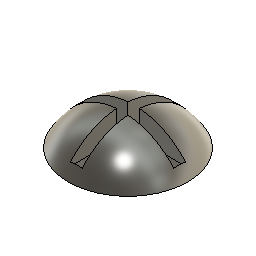
Screwhead (Autodesk Fusion 360 design; units mm, degrees)
Autodesk Fusion 360 part; units mm, degrees
sphere "SpherePrimitive1" add diameter 60 placed x (1, 0, 0) y (0, 1, 0) z (0, 0, 1) at (0, 0, 0)
sketch "Sketch2" plane through (0, 0, 0) normal (0, 0, 1) x (1, 0, 0)
  line L0 (22.5, 2.5) -> (22.5, -2.5)
  line L1 (2.5, 22.5) -> (-2.5, 22.5)
  line L2 (-22.5, 2.5) -> (-22.5, -2.5)
  line L3 (2.5, -22.5) -> (-2.5, -22.5)
  line L4 (-2.5, 22.5) -> (-2.5, 2.5)
  line L5 (-2.5, -2.5) -> (-2.5, -22.5)
  line L6 (-22.5, 2.5) -> (-2.5, 2.5)
  line L7 (2.5, 2.5) -> (22.5, 2.5)
  line L8 (2.5, 22.5) -> (2.5, 2.5)
  line L9 (2.5, -2.5) -> (2.5, -22.5)
  line L10 (-22.5, -2.5) -> (-2.5, -2.5)
  line L11 (2.5, -2.5) -> (22.5, -2.5)
  constraint collinear L4 L5
  constraint collinear L6 L7
  constraint coincident L9.start L10
  constraint collinear L8 L9
  constraint collinear L10 L11
extrude "Extrude1" cut sketch "Sketch2" along normal blind 45
sketch "Sketch3" plane through (0, -2.5, 0) normal (0, 1, 0) x (-1, 0, 0)
  arc A0 (-2.5, 29.7909) -> (-22.5, 19.685) centre (0, 0) ccw
  line L0 (-22.5, 19.685) -> (-22.5, 0)
  line L1 (-22.5, 0) -> (-2.5, 0)
  line L2 (-2.5, 0) -> (-2.5, 29.7909)
  line L3 (35, 15, -75) -> (-53.3891, 15, -75)
  line L4 (-53.3891, 15, -75) -> (-53.3891, -53.8167, -75)
  line L5 (-53.3891, -53.8167, -75) -> (35, -53.8167, -75)
  line L6 (35, -53.8167, -75) -> (35, 15, -75)
extrude "Extrude2" cut sketch "Sketch3" along normal blind 230 contours L3 L4 L5 L6 in plane through (0, -77.5, 0) normal (0, 1, 0)
sketch "Sketch4" plane through (0, 0, 15) normal (0, 0, -1) x (1, 0, 0)
  line L0 (2.5, -22.5) -> (-2.5, -22.5)
  line L1 (-2.5, -22.5) -> (-2.5, -2.5)
  line L2 (-2.5, -2.5) -> (-22.5, -2.5)
  line L3 (-22.5, -2.5) -> (-22.5, 2.5)
  line L4 (-22.5, 2.5) -> (-2.5, 2.5)
  line L5 (-2.5, 2.5) -> (-2.5, 22.5)
  line L6 (-2.5, 22.5) -> (2.5, 22.5)
  line L7 (2.5, 22.5) -> (2.5, 2.5)
  line L8 (2.5, 2.5) -> (22.5, 2.5)
  line L9 (22.5, 2.5) -> (22.5, -2.5)
  line L10 (22.5, -2.5) -> (2.5, -2.5)
  line L11 (2.5, -2.5) -> (2.5, -22.5)
  circle A0 centre (0, 0) radius 25.9808
  circle A1 centre (0, 0) radius 25.9808
  constraint coincident A0.centre A1.centre
extrude "Extrude3" add sketch "Sketch4" against normal blind 3 contours L0 L1 L2 L3 L4 L5 L6 L7 L8 L9 L10 L11
sketch "Sketch5" plane through (0, 0, 0) normal (0, 0, 1) x (1, 0, 0)
scale "Scale1" factor 0.65 about (2.5, 2.5, 18) bodies 1
sketch "Sketch6" plane through (0, 0, 0) normal (0, 1, 0) x (1, 0, 0)
